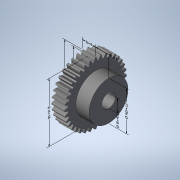
# Autodesk Inventor part: 29103600
Saved by Autodesk Inventor 2021 (Build 250183000, 183)
## iProperties
Created: 2026-04-15
Part Number: 29103600
Material: Generic
Catalog Web Link: www.3dfindit.com
Description: MAE-STZR-M0.5-POM-WS-Spur Gears Made from POM white, with One-Sided Hub, Module 0.5, Tooth Width 4 mm
Vendor: MAEDLER
Document SubType Name: Modeling
Designer: psAdmin
Manufacturer: MAEDLER
Mass: 1.8 g
Surface Area: 11.736 cm^2
Volume: 1.36263 cm^3
Density: 1 g/cm^3
Appearance: PSOLRGB-255-255-255
Category: PARTsolutions
Company: MAEDLER
Title: 29103600
Author: Cadenas PARTsolutions
Comments: Spur Gears Made from POM white, with One-Sided Hub, Module 0.5, Tooth Width 4 mm
PSOL_IDENT_0: {$CADENAS_DATA/23d-libs/maedler/antriebselemente/stirnzahnraeder/stirnzahnraeder_pom/stzr_pom_m_0_5.
PSOL_IDENT_1: prj},171 {VTYP=3D},{NB=29103600},{LINA=29103600},{NN=MAE-STZR-M0.5-POM-WS},{DATE=15.03.2026 14:49:43
PSOL_IDENT_2: },{GEOMDATE=15.03.2026 14:49:00},{VERSION=},{LINEID=220},{WBVAR=},{WBNUMERIC=}  {NB=29103600},{LINA=
PSOL_IDENT_3: 29103600},{KT=DUMMY},{ARTNR=29103600},{WEBSHOP=Produktdetails / Katalogseite / Montageanleitung},{MA
PSOL_IDENT_4: TK=Kunststoff weiß},{MAT=POM weiß},{M=0.5},{Z=36},{B=4},{DA=19.0},{D=18.0},{NL=4},{ND=12.0},{BJS10=4
PSOL_IDENT_5: },{MD=10.0},{GEW=1.80},{CTN=84839089},{DIST=0.900},{GKD=16.91447},{FKD=16.83300},{T0=1.57080},{UF=56
PSOL_IDENT_6: .54867},{TLG=1.57080},{A=3.07818},{A3=1.02606},{PI=0.39270},{R2=0.04},{CNSDWTEMPLATE=_dw/ansicht_rig
PSOL_IDENT_7: ht_front.dw}
NB: 29103600
NN: MAE-STZR-M0.5-POM-WS
NT: Spur Gears Made from POM white, with One-Sided Hub, Module 0.5, Tooth Width 4 mm
NBSYN: $ARTNR.
LINA: 29103600
CATALOG: MÄDLER
ARTNR: 29103600
WEBSHOP: Product details / Catalogue page / Assembly instructions
MATK: Plastic white
MAT: POM white
M: 0.5
Z: 36
B: 4
DA: 19
D: 18
NL: 4
ND: 12
BJS10: 4
MD: 10
GEW: 1.8
CTN: 84839089
SUPPLIER: MAEDLER
ARTICLENO: 29103600
BOMINFO: 29103600
CREATOR: CADENAS GmbH
Autodesk Inventor part; units mm, degrees
ref_plane "YZ Plane" through (0, 0, 0) normal (1, 0, 0) x (0, 1, 0)
ref_plane "XZ Plane" through (0, 0, 0) normal (0, 1, 0) x (-1, 0, 0)
ref_plane "XY Plane" through (0, 0, 0) normal (0, 0, 1) x (1, 0, 0)
sketch "Sketch_2" plane through (0, 0, 0) normal (0, 0, 1) x (1, 0, 0)
  line L0 (6, 0) -> (-2, 0)
  line L1 (-2, 9.5) -> (-2, 2.0707)
  line L2 (-2, 2.0707) -> (-1.9293, 2)
  line L3 (-1.9293, 2) -> (5.9293, 2)
  line L4 (5.9293, 2) -> (6, 2.0707)
  line L5 (6, 2.0707) -> (6, 5.9293)
  line L6 (6, 5.9293) -> (5.9293, 6)
  line L7 (5.9293, 6) -> (2.1, 6)
  arc A0 (2, 6.1) -> (2.1, 6) centre (2.1, 6.1) ccw
  line L8 (2, 6.1) -> (2, 9.5)
  line L9 (2, 9.5) -> (-2, 9.5)
  constraints: 20 end point, 2 point on circle, 1 centre point
revolve "Revolution1" add sketch "Sketch_2" angle 360 about axis through (6, 0, 0) along (1, 0, 0)
sketch "Sketch_4" plane through (0, 0, 0) normal (1, 0, 0) x (0, 0, -1)
  circle A0 centre (0, 0) radius 19
  arc A1 (-9.4982, 0.186) -> (-9.4982, -0.186) centre (0, 0) ccw
  arc A2 (-9.4982, -0.186) -> (-9.1353, -0.3433) centre (-7.9391, 2.9148) ccw
  arc A3 (-9.1353, -0.3433) -> (-8.9914, -0.3926) centre (-8.0658, 2.5431) ccw
  arc A4 (-8.9914, -0.3926) -> (-8.4349, -0.507) centre (-8.1752, 2.166) ccw
  arc A5 (-8.3989, -0.5443) -> (-8.4349, -0.507) centre (-8.4388, -0.5468) ccw
  arc A6 (-8.3989, -0.5443) -> (-8.3658, -0.9225) centre (0, 0) ccw
  arc A7 (-8.3948, -0.9654) -> (-8.3658, -0.9225) centre (-8.4056, -0.9268) ccw
  arc A8 (-8.3948, -0.9654) -> (-8.923, -1.1747) centre (-7.6749, -3.5527) ccw
  arc A9 (-8.923, -1.1747) -> (-9.0561, -1.2483) centre (-7.5017, -3.9051) ccw
  arc A10 (-9.0561, -1.2483) -> (-9.3862, -1.4661) centre (-7.3123, -4.2491) ccw
  arc A11 (-9.3862, -1.4661) -> (-9.3216, -1.8326) centre (0, 0) ccw
  arc A12 (-9.3216, -1.8326) -> (-8.9369, -1.9244) centre (-8.3246, 1.4919) ccw
  arc A13 (-8.9369, -1.9244) -> (-8.7867, -1.948) centre (-8.3849, 1.1039) ccw
  arc A14 (-8.7867, -1.948) -> (-8.2187, -1.964) centre (-8.4271, 0.7135) ccw
  arc A15 (-8.1768, -1.9944) -> (-8.2187, -1.964) centre (-8.2156, -2.0039) ccw
  arc A16 (-8.1768, -1.9944) -> (-8.0785, -2.3611) centre (0, 0) ccw
  arc A17 (-8.0997, -2.4085) -> (-8.0785, -2.3611) centre (-8.1169, -2.3724) ccw
  arc A18 (-8.0997, -2.4085) -> (-8.5835, -2.7064) centre (-6.9413, -4.8314) ccw
  arc A19 (-8.5835, -2.7064) -> (-8.7018, -2.8019) centre (-6.7096, -5.1484) ccw
  arc A20 (-8.7018, -2.8019) -> (-8.989, -3.0737) centre (-6.4633, -5.4544) ccw
  arc A21 (-8.989, -3.0737) -> (-8.8617, -3.4234) centre (0, 0) ccw
  arc A22 (-8.8617, -3.4234) -> (-8.4669, -3.447) centre (-8.4572, 0.0237) ccw
  arc A23 (-8.4669, -3.447) -> (-8.3149, -3.4442) centre (-8.4492, -0.3689) ccw
  arc A24 (-8.3149, -3.4442) -> (-7.7528, -3.3614) centre (-8.423, -0.7607) ccw
  arc A25 (-7.7062, -3.384) -> (-7.7528, -3.3614) centre (-7.7428, -3.4001) ccw
  arc A26 (-7.7062, -3.384) -> (-7.5458, -3.7281) centre (0, 0) ccw
  arc A27 (-7.5584, -3.7784) -> (-7.5458, -3.7281) centre (-7.5816, -3.7458) ccw
  arc A28 (-7.5584, -3.7784) -> (-7.9831, -4.1557) centre (-5.9969, -5.9634) ccw
  arc A29 (-7.9831, -4.1557) -> (-8.083, -4.2703) centre (-5.7136, -6.2353) ccw
  arc A30 (-8.083, -4.2703) -> (-8.3187, -4.588) centre (-5.418, -6.4938) ccw
  arc A31 (-8.3187, -4.588) -> (-8.1326, -4.9102) centre (0, 0) ccw
  arc A32 (-8.1326, -4.9102) -> (-7.7397, -4.8649) centre (-8.3328, -1.4452) ccw
  arc A33 (-7.7397, -4.8649) -> (-7.5905, -4.8357) centre (-8.2568, -1.8305) ccw
  arc A34 (-7.5905, -4.8357) -> (-7.0513, -4.6566) centre (-8.1629, -2.2118) ccw
  arc A35 (-7.0015, -4.6708) -> (-7.0513, -4.6566) centre (-7.0348, -4.693) ccw
  arc A36 (-7.0015, -4.6708) -> (-6.7838, -4.9818) centre (0, 0) ccw
  arc A37 (-6.7874, -5.0335) -> (-6.7838, -4.9818) centre (-6.816, -5.0054) ccw
  arc A38 (-6.7874, -5.0335) -> (-7.1402, -5.4789) centre (-4.8703, -6.9141) ccw
  arc A39 (-7.1402, -5.4789) -> (-7.2187, -5.6091) centre (-4.5441, -7.1328) ccw
  arc A40 (-7.2187, -5.6091) -> (-7.3956, -5.9628) centre (-4.2081, -7.336) ccw
  arc A41 (-7.3956, -5.9628) -> (-7.1564, -6.2478) centre (0, 0) ccw
  arc A42 (-7.1564, -6.2478) -> (-6.7774, -6.135) centre (-7.9553, -2.8702) ccw
  arc A43 (-6.7774, -6.135) -> (-6.6355, -6.0803) centre (-7.8135, -3.2364) ccw
  arc A44 (-6.6355, -6.0803) -> (-6.1356, -5.8103) centre (-7.6548, -3.5957) ccw
  arc A45 (-6.0841, -5.8156) -> (-6.1356, -5.8103) centre (-6.113, -5.8433) ccw
  arc A46 (-6.0841, -5.8156) -> (-5.8156, -6.0841) centre (0, 0) ccw
  arc A47 (-5.8103, -6.1356) -> (-5.8156, -6.0841) centre (-5.8433, -6.113) ccw
  arc A48 (-5.8103, -6.1356) -> (-6.0803, -6.6355) centre (-3.5957, -7.6548) ccw
  arc A49 (-6.0803, -6.6355) -> (-6.135, -6.7774) centre (-3.2364, -7.8135) ccw
  arc A50 (-6.135, -6.7774) -> (-6.2478, -7.1564) centre (-2.8702, -7.9553) ccw
  arc A51 (-6.2478, -7.1564) -> (-5.9628, -7.3956) centre (0, 0) ccw
  arc A52 (-5.9628, -7.3956) -> (-5.6091, -7.2187) centre (-7.336, -4.2081) ccw
  arc A53 (-5.6091, -7.2187) -> (-5.4789, -7.1402) centre (-7.1328, -4.5441) ccw
  arc A54 (-5.4789, -7.1402) -> (-5.0335, -6.7874) centre (-6.9141, -4.8703) ccw
  arc A55 (-4.9818, -6.7838) -> (-5.0335, -6.7874) centre (-5.0054, -6.816) ccw
  arc A56 (-4.9818, -6.7838) -> (-4.6708, -7.0015) centre (0, 0) ccw
  arc A57 (-4.6566, -7.0513) -> (-4.6708, -7.0015) centre (-4.693, -7.0348) ccw
  arc A58 (-4.6566, -7.0513) -> (-4.8357, -7.5905) centre (-2.2118, -8.1629) ccw
  arc A59 (-4.8357, -7.5905) -> (-4.8649, -7.7397) centre (-1.8305, -8.2568) ccw
  arc A60 (-4.8649, -7.7397) -> (-4.9102, -8.1326) centre (-1.4452, -8.3328) ccw
  arc A61 (-4.9102, -8.1326) -> (-4.588, -8.3187) centre (0, 0) ccw
  arc A62 (-4.588, -8.3187) -> (-4.2703, -8.083) centre (-6.4938, -5.418) ccw
  arc A63 (-4.2703, -8.083) -> (-4.1557, -7.9831) centre (-6.2353, -5.7136) ccw
  arc A64 (-4.1557, -7.9831) -> (-3.7784, -7.5584) centre (-5.9634, -5.9969) ccw
  arc A65 (-3.7281, -7.5458) -> (-3.7784, -7.5584) centre (-3.7458, -7.5816) ccw
  arc A66 (-3.7281, -7.5458) -> (-3.384, -7.7062) centre (0, 0) ccw
  arc A67 (-3.3614, -7.7528) -> (-3.384, -7.7062) centre (-3.4001, -7.7428) ccw
  arc A68 (-3.3614, -7.7528) -> (-3.4442, -8.3149) centre (-0.7607, -8.423) ccw
  arc A69 (-3.4442, -8.3149) -> (-3.447, -8.4669) centre (-0.3689, -8.4492) ccw
  arc A70 (-3.447, -8.4669) -> (-3.4234, -8.8617) centre (0.0237, -8.4572) ccw
  arc A71 (-3.4234, -8.8617) -> (-3.0737, -8.989) centre (0, 0) ccw
  arc A72 (-3.0737, -8.989) -> (-2.8019, -8.7018) centre (-5.4544, -6.4633) ccw
  arc A73 (-2.8019, -8.7018) -> (-2.7064, -8.5835) centre (-5.1484, -6.7096) ccw
  arc A74 (-2.7064, -8.5835) -> (-2.4085, -8.0997) centre (-4.8314, -6.9413) ccw
  arc A75 (-2.3611, -8.0785) -> (-2.4085, -8.0997) centre (-2.3724, -8.1169) ccw
  arc A76 (-2.3611, -8.0785) -> (-1.9944, -8.1768) centre (0, 0) ccw
  arc A77 (-1.964, -8.2187) -> (-1.9944, -8.1768) centre (-2.0039, -8.2156) ccw
  arc A78 (-1.964, -8.2187) -> (-1.948, -8.7867) centre (0.7135, -8.4271) ccw
  arc A79 (-1.948, -8.7867) -> (-1.9244, -8.9369) centre (1.1039, -8.3849) ccw
  arc A80 (-1.9244, -8.9369) -> (-1.8326, -9.3216) centre (1.4919, -8.3246) ccw
  arc A81 (-1.8326, -9.3216) -> (-1.4661, -9.3862) centre (0, 0) ccw
  arc A82 (-1.4661, -9.3862) -> (-1.2483, -9.0561) centre (-4.2491, -7.3123) ccw
  arc A83 (-1.2483, -9.0561) -> (-1.1747, -8.923) centre (-3.9051, -7.5017) ccw
  arc A84 (-1.1747, -8.923) -> (-0.9654, -8.3948) centre (-3.5527, -7.6749) ccw
  arc A85 (-0.9225, -8.3658) -> (-0.9654, -8.3948) centre (-0.9268, -8.4056) ccw
  arc A86 (-0.9225, -8.3658) -> (-0.5443, -8.3989) centre (0, 0) ccw
  arc A87 (-0.507, -8.4349) -> (-0.5443, -8.3989) centre (-0.5468, -8.4388) ccw
  arc A88 (-0.507, -8.4349) -> (-0.3926, -8.9914) centre (2.166, -8.1752) ccw
  arc A89 (-0.3926, -8.9914) -> (-0.3433, -9.1353) centre (2.5431, -8.0658) ccw
  arc A90 (-0.3433, -9.1353) -> (-0.186, -9.4982) centre (2.9148, -7.9391) ccw
  arc A91 (-0.186, -9.4982) -> (0.186, -9.4982) centre (0, 0) ccw
  arc A92 (0.186, -9.4982) -> (0.3433, -9.1353) centre (-2.9148, -7.9391) ccw
  arc A93 (0.3433, -9.1353) -> (0.3926, -8.9914) centre (-2.5431, -8.0658) ccw
  arc A94 (0.3926, -8.9914) -> (0.507, -8.4349) centre (-2.166, -8.1752) ccw
  arc A95 (0.5443, -8.3989) -> (0.507, -8.4349) centre (0.5468, -8.4388) ccw
  arc A96 (0.5443, -8.3989) -> (0.9225, -8.3658) centre (0, 0) ccw
  arc A97 (0.9654, -8.3948) -> (0.9225, -8.3658) centre (0.9268, -8.4056) ccw
  arc A98 (0.9654, -8.3948) -> (1.1747, -8.923) centre (3.5527, -7.6749) ccw
  arc A99 (1.1747, -8.923) -> (1.2483, -9.0561) centre (3.9051, -7.5017) ccw
  arc A100 (1.2483, -9.0561) -> (1.4661, -9.3862) centre (4.2491, -7.3123) ccw
  arc A101 (1.4661, -9.3862) -> (1.8326, -9.3216) centre (0, 0) ccw
  arc A102 (1.8326, -9.3216) -> (1.9244, -8.9369) centre (-1.4919, -8.3246) ccw
  arc A103 (1.9244, -8.9369) -> (1.948, -8.7867) centre (-1.1039, -8.3849) ccw
  arc A104 (1.948, -8.7867) -> (1.964, -8.2187) centre (-0.7135, -8.4271) ccw
  arc A105 (1.9944, -8.1768) -> (1.964, -8.2187) centre (2.0039, -8.2156) ccw
  arc A106 (1.9944, -8.1768) -> (2.3611, -8.0785) centre (0, 0) ccw
  arc A107 (2.4085, -8.0997) -> (2.3611, -8.0785) centre (2.3724, -8.1169) ccw
  arc A108 (2.4085, -8.0997) -> (2.7064, -8.5835) centre (4.8314, -6.9413) ccw
  arc A109 (2.7064, -8.5835) -> (2.8019, -8.7018) centre (5.1484, -6.7096) ccw
  arc A110 (2.8019, -8.7018) -> (3.0737, -8.989) centre (5.4544, -6.4633) ccw
  arc A111 (3.0737, -8.989) -> (3.4234, -8.8617) centre (0, 0) ccw
  arc A112 (3.4234, -8.8617) -> (3.447, -8.4669) centre (-0.0237, -8.4572) ccw
  arc A113 (3.447, -8.4669) -> (3.4442, -8.3149) centre (0.3689, -8.4492) ccw
  arc A114 (3.4442, -8.3149) -> (3.3614, -7.7528) centre (0.7607, -8.423) ccw
  arc A115 (3.384, -7.7062) -> (3.3614, -7.7528) centre (3.4001, -7.7428) ccw
  arc A116 (3.384, -7.7062) -> (3.7281, -7.5458) centre (0, 0) ccw
  arc A117 (3.7784, -7.5584) -> (3.7281, -7.5458) centre (3.7458, -7.5816) ccw
  arc A118 (3.7784, -7.5584) -> (4.1557, -7.9831) centre (5.9634, -5.9969) ccw
  arc A119 (4.1557, -7.9831) -> (4.2703, -8.083) centre (6.2353, -5.7136) ccw
  arc A120 (4.2703, -8.083) -> (4.588, -8.3187) centre (6.4938, -5.418) ccw
  arc A121 (4.588, -8.3187) -> (4.9102, -8.1326) centre (0, 0) ccw
  arc A122 (4.9102, -8.1326) -> (4.8649, -7.7397) centre (1.4452, -8.3328) ccw
  arc A123 (4.8649, -7.7397) -> (4.8357, -7.5905) centre (1.8305, -8.2568) ccw
  arc A124 (4.8357, -7.5905) -> (4.6566, -7.0513) centre (2.2118, -8.1629) ccw
  arc A125 (4.6708, -7.0015) -> (4.6566, -7.0513) centre (4.693, -7.0348) ccw
  arc A126 (4.6708, -7.0015) -> (4.9818, -6.7838) centre (0, 0) ccw
  arc A127 (5.0335, -6.7874) -> (4.9818, -6.7838) centre (5.0054, -6.816) ccw
  arc A128 (5.0335, -6.7874) -> (5.4789, -7.1402) centre (6.9141, -4.8703) ccw
  arc A129 (5.4789, -7.1402) -> (5.6091, -7.2187) centre (7.1328, -4.5441) ccw
  arc A130 (5.6091, -7.2187) -> (5.9628, -7.3956) centre (7.336, -4.2081) ccw
  arc A131 (5.9628, -7.3956) -> (6.2478, -7.1564) centre (0, 0) ccw
  arc A132 (6.2478, -7.1564) -> (6.135, -6.7774) centre (2.8702, -7.9553) ccw
  arc A133 (6.135, -6.7774) -> (6.0803, -6.6355) centre (3.2364, -7.8135) ccw
  arc A134 (6.0803, -6.6355) -> (5.8103, -6.1356) centre (3.5957, -7.6548) ccw
  arc A135 (5.8156, -6.0841) -> (5.8103, -6.1356) centre (5.8433, -6.113) ccw
  arc A136 (5.8156, -6.0841) -> (6.0841, -5.8156) centre (0, 0) ccw
  arc A137 (6.1356, -5.8103) -> (6.0841, -5.8156) centre (6.113, -5.8433) ccw
  arc A138 (6.1356, -5.8103) -> (6.6355, -6.0803) centre (7.6548, -3.5957) ccw
  arc A139 (6.6355, -6.0803) -> (6.7774, -6.135) centre (7.8135, -3.2364) ccw
  arc A140 (6.7774, -6.135) -> (7.1564, -6.2478) centre (7.9553, -2.8702) ccw
  arc A141 (7.1564, -6.2478) -> (7.3956, -5.9628) centre (0, 0) ccw
  arc A142 (7.3956, -5.9628) -> (7.2187, -5.6091) centre (4.2081, -7.336) ccw
  arc A143 (7.2187, -5.6091) -> (7.1402, -5.4789) centre (4.5441, -7.1328) ccw
  arc A144 (7.1402, -5.4789) -> (6.7874, -5.0335) centre (4.8703, -6.9141) ccw
  arc A145 (6.7838, -4.9818) -> (6.7874, -5.0335) centre (6.816, -5.0054) ccw
  arc A146 (6.7838, -4.9818) -> (7.0015, -4.6708) centre (0, 0) ccw
  arc A147 (7.0513, -4.6566) -> (7.0015, -4.6708) centre (7.0348, -4.693) ccw
  arc A148 (7.0513, -4.6566) -> (7.5905, -4.8357) centre (8.1629, -2.2118) ccw
  arc A149 (7.5905, -4.8357) -> (7.7397, -4.8649) centre (8.2568, -1.8305) ccw
  arc A150 (7.7397, -4.8649) -> (8.1326, -4.9102) centre (8.3328, -1.4452) ccw
  arc A151 (8.1326, -4.9102) -> (8.3187, -4.588) centre (0, 0) ccw
  arc A152 (8.3187, -4.588) -> (8.083, -4.2703) centre (5.418, -6.4938) ccw
  arc A153 (8.083, -4.2703) -> (7.9831, -4.1557) centre (5.7136, -6.2353) ccw
  arc A154 (7.9831, -4.1557) -> (7.5584, -3.7784) centre (5.9969, -5.9634) ccw
  arc A155 (7.5458, -3.7281) -> (7.5584, -3.7784) centre (7.5816, -3.7458) ccw
  arc A156 (7.5458, -3.7281) -> (7.7062, -3.384) centre (0, 0) ccw
  arc A157 (7.7528, -3.3614) -> (7.7062, -3.384) centre (7.7428, -3.4001) ccw
  arc A158 (7.7528, -3.3614) -> (8.3149, -3.4442) centre (8.423, -0.7607) ccw
  arc A159 (8.3149, -3.4442) -> (8.4669, -3.447) centre (8.4492, -0.3689) ccw
  arc A160 (8.4669, -3.447) -> (8.8617, -3.4234) centre (8.4572, 0.0237) ccw
  arc A161 (8.8617, -3.4234) -> (8.989, -3.0737) centre (0, 0) ccw
  arc A162 (8.989, -3.0737) -> (8.7018, -2.8019) centre (6.4633, -5.4544) ccw
  arc A163 (8.7018, -2.8019) -> (8.5835, -2.7064) centre (6.7096, -5.1484) ccw
  arc A164 (8.5835, -2.7064) -> (8.0997, -2.4085) centre (6.9413, -4.8314) ccw
  arc A165 (8.0785, -2.3611) -> (8.0997, -2.4085) centre (8.1169, -2.3724) ccw
  arc A166 (8.0785, -2.3611) -> (8.1768, -1.9944) centre (0, 0) ccw
  arc A167 (8.2187, -1.964) -> (8.1768, -1.9944) centre (8.2156, -2.0039) ccw
  arc A168 (8.2187, -1.964) -> (8.7867, -1.948) centre (8.4271, 0.7135) ccw
  arc A169 (8.7867, -1.948) -> (8.9369, -1.9244) centre (8.3849, 1.1039) ccw
  arc A170 (8.9369, -1.9244) -> (9.3216, -1.8326) centre (8.3246, 1.4919) ccw
  arc A171 (9.3216, -1.8326) -> (9.3862, -1.4661) centre (0, 0) ccw
  arc A172 (9.3862, -1.4661) -> (9.0561, -1.2483) centre (7.3123, -4.2491) ccw
  arc A173 (9.0561, -1.2483) -> (8.923, -1.1747) centre (7.5017, -3.9051) ccw
  arc A174 (8.923, -1.1747) -> (8.3948, -0.9654) centre (7.6749, -3.5527) ccw
  arc A175 (8.3658, -0.9225) -> (8.3948, -0.9654) centre (8.4056, -0.9268) ccw
  arc A176 (8.3658, -0.9225) -> (8.3989, -0.5443) centre (0, 0) ccw
  arc A177 (8.4349, -0.507) -> (8.3989, -0.5443) centre (8.4388, -0.5468) ccw
  arc A178 (8.4349, -0.507) -> (8.9914, -0.3926) centre (8.1752, 2.166) ccw
  arc A179 (8.9914, -0.3926) -> (9.1353, -0.3433) centre (8.0658, 2.5431) ccw
  arc A180 (9.1353, -0.3433) -> (9.4982, -0.186) centre (7.9391, 2.9148) ccw
  arc A181 (9.4982, -0.186) -> (9.4982, 0.186) centre (0, 0) ccw
  arc A182 (9.4982, 0.186) -> (9.1353, 0.3433) centre (7.9391, -2.9148) ccw
  arc A183 (9.1353, 0.3433) -> (8.9914, 0.3926) centre (8.0658, -2.5431) ccw
  arc A184 (8.9914, 0.3926) -> (8.4349, 0.507) centre (8.1752, -2.166) ccw
  arc A185 (8.3989, 0.5443) -> (8.4349, 0.507) centre (8.4388, 0.5468) ccw
  arc A186 (8.3989, 0.5443) -> (8.3658, 0.9225) centre (0, 0) ccw
  arc A187 (8.3948, 0.9654) -> (8.3658, 0.9225) centre (8.4056, 0.9268) ccw
  arc A188 (8.3948, 0.9654) -> (8.923, 1.1747) centre (7.6749, 3.5527) ccw
  arc A189 (8.923, 1.1747) -> (9.0561, 1.2483) centre (7.5017, 3.9051) ccw
  arc A190 (9.0561, 1.2483) -> (9.3862, 1.4661) centre (7.3123, 4.2491) ccw
  arc A191 (9.3862, 1.4661) -> (9.3216, 1.8326) centre (0, 0) ccw
  arc A192 (9.3216, 1.8326) -> (8.9369, 1.9244) centre (8.3246, -1.4919) ccw
  arc A193 (8.9369, 1.9244) -> (8.7867, 1.948) centre (8.3849, -1.1039) ccw
  arc A194 (8.7867, 1.948) -> (8.2187, 1.964) centre (8.4271, -0.7135) ccw
  arc A195 (8.1768, 1.9944) -> (8.2187, 1.964) centre (8.2156, 2.0039) ccw
  arc A196 (8.1768, 1.9944) -> (8.0785, 2.3611) centre (0, 0) ccw
  arc A197 (8.0997, 2.4085) -> (8.0785, 2.3611) centre (8.1169, 2.3724) ccw
  arc A198 (8.0997, 2.4085) -> (8.5835, 2.7064) centre (6.9413, 4.8314) ccw
  arc A199 (8.5835, 2.7064) -> (8.7018, 2.8019) centre (6.7096, 5.1484) ccw
  arc A200 (8.7018, 2.8019) -> (8.989, 3.0737) centre (6.4633, 5.4544) ccw
  arc A201 (8.989, 3.0737) -> (8.8617, 3.4234) centre (0, 0) ccw
  arc A202 (8.8617, 3.4234) -> (8.4669, 3.447) centre (8.4572, -0.0237) ccw
  arc A203 (8.4669, 3.447) -> (8.3149, 3.4442) centre (8.4492, 0.3689) ccw
  arc A204 (8.3149, 3.4442) -> (7.7528, 3.3614) centre (8.423, 0.7607) ccw
  arc A205 (7.7062, 3.384) -> (7.7528, 3.3614) centre (7.7428, 3.4001) ccw
  arc A206 (7.7062, 3.384) -> (7.5458, 3.7281) centre (0, 0) ccw
  arc A207 (7.5584, 3.7784) -> (7.5458, 3.7281) centre (7.5816, 3.7458) ccw
  arc A208 (7.5584, 3.7784) -> (7.9831, 4.1557) centre (5.9969, 5.9634) ccw
  arc A209 (7.9831, 4.1557) -> (8.083, 4.2703) centre (5.7136, 6.2353) ccw
  arc A210 (8.083, 4.2703) -> (8.3187, 4.588) centre (5.418, 6.4938) ccw
  arc A211 (8.3187, 4.588) -> (8.1326, 4.9102) centre (0, 0) ccw
  arc A212 (8.1326, 4.9102) -> (7.7397, 4.8649) centre (8.3328, 1.4452) ccw
  arc A213 (7.7397, 4.8649) -> (7.5905, 4.8357) centre (8.2568, 1.8305) ccw
  arc A214 (7.5905, 4.8357) -> (7.0513, 4.6566) centre (8.1629, 2.2118) ccw
  arc A215 (7.0015, 4.6708) -> (7.0513, 4.6566) centre (7.0348, 4.693) ccw
  arc A216 (7.0015, 4.6708) -> (6.7838, 4.9818) centre (0, 0) ccw
  arc A217 (6.7874, 5.0335) -> (6.7838, 4.9818) centre (6.816, 5.0054) ccw
  arc A218 (6.7874, 5.0335) -> (7.1402, 5.4789) centre (4.8703, 6.9141) ccw
  arc A219 (7.1402, 5.4789) -> (7.2187, 5.6091) centre (4.5441, 7.1328) ccw
  arc A220 (7.2187, 5.6091) -> (7.3956, 5.9628) centre (4.2081, 7.336) ccw
  arc A221 (7.3956, 5.9628) -> (7.1564, 6.2478) centre (0, 0) ccw
  arc A222 (7.1564, 6.2478) -> (6.7774, 6.135) centre (7.9553, 2.8702) ccw
  arc A223 (6.7774, 6.135) -> (6.6355, 6.0803) centre (7.8135, 3.2364) ccw
  arc A224 (6.6355, 6.0803) -> (6.1356, 5.8103) centre (7.6548, 3.5957) ccw
  arc A225 (6.0841, 5.8156) -> (6.1356, 5.8103) centre (6.113, 5.8433) ccw
  arc A226 (6.0841, 5.8156) -> (5.8156, 6.0841) centre (0, 0) ccw
  arc A227 (5.8103, 6.1356) -> (5.8156, 6.0841) centre (5.8433, 6.113) ccw
  arc A228 (5.8103, 6.1356) -> (6.0803, 6.6355) centre (3.5957, 7.6548) ccw
  arc A229 (6.0803, 6.6355) -> (6.135, 6.7774) centre (3.2364, 7.8135) ccw
  arc A230 (6.135, 6.7774) -> (6.2478, 7.1564) centre (2.8702, 7.9553) ccw
  arc A231 (6.2478, 7.1564) -> (5.9628, 7.3956) centre (0, 0) ccw
  arc A232 (5.9628, 7.3956) -> (5.6091, 7.2187) centre (7.336, 4.2081) ccw
  arc A233 (5.6091, 7.2187) -> (5.4789, 7.1402) centre (7.1328, 4.5441) ccw
  arc A234 (5.4789, 7.1402) -> (5.0335, 6.7874) centre (6.9141, 4.8703) ccw
  arc A235 (4.9818, 6.7838) -> (5.0335, 6.7874) centre (5.0054, 6.816) ccw
  arc A236 (4.9818, 6.7838) -> (4.6708, 7.0015) centre (0, 0) ccw
  arc A237 (4.6566, 7.0513) -> (4.6708, 7.0015) centre (4.693, 7.0348) ccw
  arc A238 (4.6566, 7.0513) -> (4.8357, 7.5905) centre (2.2118, 8.1629) ccw
  arc A239 (4.8357, 7.5905) -> (4.8649, 7.7397) centre (1.8305, 8.2568) ccw
  arc A240 (4.8649, 7.7397) -> (4.9102, 8.1326) centre (1.4452, 8.3328) ccw
  arc A241 (4.9102, 8.1326) -> (4.588, 8.3187) centre (0, 0) ccw
  arc A242 (4.588, 8.3187) -> (4.2703, 8.083) centre (6.4938, 5.418) ccw
  arc A243 (4.2703, 8.083) -> (4.1557, 7.9831) centre (6.2353, 5.7136) ccw
  arc A244 (4.1557, 7.9831) -> (3.7784, 7.5584) centre (5.9634, 5.9969) ccw
  arc A245 (3.7281, 7.5458) -> (3.7784, 7.5584) centre (3.7458, 7.5816) ccw
  arc A246 (3.7281, 7.5458) -> (3.384, 7.7062) centre (0, 0) ccw
  arc A247 (3.3614, 7.7528) -> (3.384, 7.7062) centre (3.4001, 7.7428) ccw
  arc A248 (3.3614, 7.7528) -> (3.4442, 8.3149) centre (0.7607, 8.423) ccw
  arc A249 (3.4442, 8.3149) -> (3.447, 8.4669) centre (0.3689, 8.4492) ccw
  arc A250 (3.447, 8.4669) -> (3.4234, 8.8617) centre (-0.0237, 8.4572) ccw
  arc A251 (3.4234, 8.8617) -> (3.0737, 8.989) centre (0, 0) ccw
  arc A252 (3.0737, 8.989) -> (2.8019, 8.7018) centre (5.4544, 6.4633) ccw
  arc A253 (2.8019, 8.7018) -> (2.7064, 8.5835) centre (5.1484, 6.7096) ccw
  arc A254 (2.7064, 8.5835) -> (2.4085, 8.0997) centre (4.8314, 6.9413) ccw
  arc A255 (2.3611, 8.0785) -> (2.4085, 8.0997) centre (2.3724, 8.1169) ccw
  arc A256 (2.3611, 8.0785) -> (1.9944, 8.1768) centre (0, 0) ccw
  arc A257 (1.964, 8.2187) -> (1.9944, 8.1768) centre (2.0039, 8.2156) ccw
  arc A258 (1.964, 8.2187) -> (1.948, 8.7867) centre (-0.7135, 8.4271) ccw
  arc A259 (1.948, 8.7867) -> (1.9244, 8.9369) centre (-1.1039, 8.3849) ccw
  arc A260 (1.9244, 8.9369) -> (1.8326, 9.3216) centre (-1.4919, 8.3246) ccw
  arc A261 (1.8326, 9.3216) -> (1.4661, 9.3862) centre (0, 0) ccw
  arc A262 (1.4661, 9.3862) -> (1.2483, 9.0561) centre (4.2491, 7.3123) ccw
  arc A263 (1.2483, 9.0561) -> (1.1747, 8.923) centre (3.9051, 7.5017) ccw
  arc A264 (1.1747, 8.923) -> (0.9654, 8.3948) centre (3.5527, 7.6749) ccw
  arc A265 (0.9225, 8.3658) -> (0.9654, 8.3948) centre (0.9268, 8.4056) ccw
  arc A266 (0.9225, 8.3658) -> (0.5443, 8.3989) centre (0, 0) ccw
  arc A267 (0.507, 8.4349) -> (0.5443, 8.3989) centre (0.5468, 8.4388) ccw
  arc A268 (0.507, 8.4349) -> (0.3926, 8.9914) centre (-2.166, 8.1752) ccw
  arc A269 (0.3926, 8.9914) -> (0.3433, 9.1353) centre (-2.5431, 8.0658) ccw
  arc A270 (0.3433, 9.1353) -> (0.186, 9.4982) centre (-2.9148, 7.9391) ccw
  arc A271 (0.186, 9.4982) -> (-0.186, 9.4982) centre (0, 0) ccw
  arc A272 (-0.186, 9.4982) -> (-0.3433, 9.1353) centre (2.9148, 7.9391) ccw
  arc A273 (-0.3433, 9.1353) -> (-0.3926, 8.9914) centre (2.5431, 8.0658) ccw
  arc A274 (-0.3926, 8.9914) -> (-0.507, 8.4349) centre (2.166, 8.1752) ccw
  arc A275 (-0.5443, 8.3989) -> (-0.507, 8.4349) centre (-0.5468, 8.4388) ccw
  arc A276 (-0.5443, 8.3989) -> (-0.9225, 8.3658) centre (0, 0) ccw
  arc A277 (-0.9654, 8.3948) -> (-0.9225, 8.3658) centre (-0.9268, 8.4056) ccw
  arc A278 (-0.9654, 8.3948) -> (-1.1747, 8.923) centre (-3.5527, 7.6749) ccw
  arc A279 (-1.1747, 8.923) -> (-1.2483, 9.0561) centre (-3.9051, 7.5017) ccw
  arc A280 (-1.2483, 9.0561) -> (-1.4661, 9.3862) centre (-4.2491, 7.3123) ccw
  arc A281 (-1.4661, 9.3862) -> (-1.8326, 9.3216) centre (0, 0) ccw
  arc A282 (-1.8326, 9.3216) -> (-1.9244, 8.9369) centre (1.4919, 8.3246) ccw
  arc A283 (-1.9244, 8.9369) -> (-1.948, 8.7867) centre (1.1039, 8.3849) ccw
  arc A284 (-1.948, 8.7867) -> (-1.964, 8.2187) centre (0.7135, 8.4271) ccw
  arc A285 (-1.9944, 8.1768) -> (-1.964, 8.2187) centre (-2.0039, 8.2156) ccw
  arc A286 (-1.9944, 8.1768) -> (-2.3611, 8.0785) centre (0, 0) ccw
  arc A287 (-2.4085, 8.0997) -> (-2.3611, 8.0785) centre (-2.3724, 8.1169) ccw
  arc A288 (-2.4085, 8.0997) -> (-2.7064, 8.5835) centre (-4.8314, 6.9413) ccw
  arc A289 (-2.7064, 8.5835) -> (-2.8019, 8.7018) centre (-5.1484, 6.7096) ccw
  arc A290 (-2.8019, 8.7018) -> (-3.0737, 8.989) centre (-5.4544, 6.4633) ccw
  arc A291 (-3.0737, 8.989) -> (-3.4234, 8.8617) centre (0, 0) ccw
  arc A292 (-3.4234, 8.8617) -> (-3.447, 8.4669) centre (0.0237, 8.4572) ccw
  arc A293 (-3.447, 8.4669) -> (-3.4442, 8.3149) centre (-0.3689, 8.4492) ccw
  arc A294 (-3.4442, 8.3149) -> (-3.3614, 7.7528) centre (-0.7607, 8.423) ccw
  arc A295 (-3.384, 7.7062) -> (-3.3614, 7.7528) centre (-3.4001, 7.7428) ccw
  arc A296 (-3.384, 7.7062) -> (-3.7281, 7.5458) centre (0, 0) ccw
  arc A297 (-3.7784, 7.5584) -> (-3.7281, 7.5458) centre (-3.7458, 7.5816) ccw
  arc A298 (-3.7784, 7.5584) -> (-4.1557, 7.9831) centre (-5.9634, 5.9969) ccw
  arc A299 (-4.1557, 7.9831) -> (-4.2703, 8.083) centre (-6.2353, 5.7136) ccw
  arc A300 (-4.2703, 8.083) -> (-4.588, 8.3187) centre (-6.4938, 5.418) ccw
  arc A301 (-4.588, 8.3187) -> (-4.9102, 8.1326) centre (0, 0) ccw
  arc A302 (-4.9102, 8.1326) -> (-4.8649, 7.7397) centre (-1.4452, 8.3328) ccw
  arc A303 (-4.8649, 7.7397) -> (-4.8357, 7.5905) centre (-1.8305, 8.2568) ccw
  arc A304 (-4.8357, 7.5905) -> (-4.6566, 7.0513) centre (-2.2118, 8.1629) ccw
  arc A305 (-4.6708, 7.0015) -> (-4.6566, 7.0513) centre (-4.693, 7.0348) ccw
  arc A306 (-4.6708, 7.0015) -> (-4.9818, 6.7838) centre (0, 0) ccw
  arc A307 (-5.0335, 6.7874) -> (-4.9818, 6.7838) centre (-5.0054, 6.816) ccw
  arc A308 (-5.0335, 6.7874) -> (-5.4789, 7.1402) centre (-6.9141, 4.8703) ccw
  arc A309 (-5.4789, 7.1402) -> (-5.6091, 7.2187) centre (-7.1328, 4.5441) ccw
  arc A310 (-5.6091, 7.2187) -> (-5.9628, 7.3956) centre (-7.336, 4.2081) ccw
  arc A311 (-5.9628, 7.3956) -> (-6.2478, 7.1564) centre (0, 0) ccw
  arc A312 (-6.2478, 7.1564) -> (-6.135, 6.7774) centre (-2.8702, 7.9553) ccw
  arc A313 (-6.135, 6.7774) -> (-6.0803, 6.6355) centre (-3.2364, 7.8135) ccw
  arc A314 (-6.0803, 6.6355) -> (-5.8103, 6.1356) centre (-3.5957, 7.6548) ccw
  arc A315 (-5.8156, 6.0841) -> (-5.8103, 6.1356) centre (-5.8433, 6.113) ccw
  arc A316 (-5.8156, 6.0841) -> (-6.0841, 5.8156) centre (0, 0) ccw
  arc A317 (-6.1356, 5.8103) -> (-6.0841, 5.8156) centre (-6.113, 5.8433) ccw
  arc A318 (-6.1356, 5.8103) -> (-6.6355, 6.0803) centre (-7.6548, 3.5957) ccw
  arc A319 (-6.6355, 6.0803) -> (-6.7774, 6.135) centre (-7.8135, 3.2364) ccw
  arc A320 (-6.7774, 6.135) -> (-7.1564, 6.2478) centre (-7.9553, 2.8702) ccw
  arc A321 (-7.1564, 6.2478) -> (-7.3956, 5.9628) centre (0, 0) ccw
  arc A322 (-7.3956, 5.9628) -> (-7.2187, 5.6091) centre (-4.2081, 7.336) ccw
  arc A323 (-7.2187, 5.6091) -> (-7.1402, 5.4789) centre (-4.5441, 7.1328) ccw
  arc A324 (-7.1402, 5.4789) -> (-6.7874, 5.0335) centre (-4.8703, 6.9141) ccw
  arc A325 (-6.7838, 4.9818) -> (-6.7874, 5.0335) centre (-6.816, 5.0054) ccw
  arc A326 (-6.7838, 4.9818) -> (-7.0015, 4.6708) centre (0, 0) ccw
  arc A327 (-7.0513, 4.6566) -> (-7.0015, 4.6708) centre (-7.0348, 4.693) ccw
  arc A328 (-7.0513, 4.6566) -> (-7.5905, 4.8357) centre (-8.1629, 2.2118) ccw
  arc A329 (-7.5905, 4.8357) -> (-7.7397, 4.8649) centre (-8.2568, 1.8305) ccw
  arc A330 (-7.7397, 4.8649) -> (-8.1326, 4.9102) centre (-8.3328, 1.4452) ccw
  arc A331 (-8.1326, 4.9102) -> (-8.3187, 4.588) centre (0, 0) ccw
  arc A332 (-8.3187, 4.588) -> (-8.083, 4.2703) centre (-5.418, 6.4938) ccw
  arc A333 (-8.083, 4.2703) -> (-7.9831, 4.1557) centre (-5.7136, 6.2353) ccw
  arc A334 (-7.9831, 4.1557) -> (-7.5584, 3.7784) centre (-5.9969, 5.9634) ccw
  arc A335 (-7.5458, 3.7281) -> (-7.5584, 3.7784) centre (-7.5816, 3.7458) ccw
  arc A336 (-7.5458, 3.7281) -> (-7.7062, 3.384) centre (0, 0) ccw
  arc A337 (-7.7528, 3.3614) -> (-7.7062, 3.384) centre (-7.7428, 3.4001) ccw
  arc A338 (-7.7528, 3.3614) -> (-8.3149, 3.4442) centre (-8.423, 0.7607) ccw
  arc A339 (-8.3149, 3.4442) -> (-8.4669, 3.447) centre (-8.4492, 0.3689) ccw
  arc A340 (-8.4669, 3.447) -> (-8.8617, 3.4234) centre (-8.4572, -0.0237) ccw
  arc A341 (-8.8617, 3.4234) -> (-8.989, 3.0737) centre (0, 0) ccw
  arc A342 (-8.989, 3.0737) -> (-8.7018, 2.8019) centre (-6.4633, 5.4544) ccw
  arc A343 (-8.7018, 2.8019) -> (-8.5835, 2.7064) centre (-6.7096, 5.1484) ccw
  arc A344 (-8.5835, 2.7064) -> (-8.0997, 2.4085) centre (-6.9413, 4.8314) ccw
  arc A345 (-8.0785, 2.3611) -> (-8.0997, 2.4085) centre (-8.1169, 2.3724) ccw
  arc A346 (-8.0785, 2.3611) -> (-8.1768, 1.9944) centre (0, 0) ccw
  arc A347 (-8.2187, 1.964) -> (-8.1768, 1.9944) centre (-8.2156, 2.0039) ccw
  arc A348 (-8.2187, 1.964) -> (-8.7867, 1.948) centre (-8.4271, -0.7135) ccw
  arc A349 (-8.7867, 1.948) -> (-8.9369, 1.9244) centre (-8.3849, -1.1039) ccw
  arc A350 (-8.9369, 1.9244) -> (-9.3216, 1.8326) centre (-8.3246, -1.4919) ccw
  arc A351 (-9.3216, 1.8326) -> (-9.3862, 1.4661) centre (0, 0) ccw
  arc A352 (-9.3862, 1.4661) -> (-9.0561, 1.2483) centre (-7.3123, 4.2491) ccw
  arc A353 (-9.0561, 1.2483) -> (-8.923, 1.1747) centre (-7.5017, 3.9051) ccw
  arc A354 (-8.923, 1.1747) -> (-8.3948, 0.9654) centre (-7.6749, 3.5527) ccw
  arc A355 (-8.3658, 0.9225) -> (-8.3948, 0.9654) centre (-8.4056, 0.9268) ccw
  arc A356 (-8.3658, 0.9225) -> (-8.3989, 0.5443) centre (0, 0) ccw
  arc A357 (-8.4349, 0.507) -> (-8.3989, 0.5443) centre (-8.4388, 0.5468) ccw
  arc A358 (-8.4349, 0.507) -> (-8.9914, 0.3926) centre (-8.1752, -2.166) ccw
  arc A359 (-8.9914, 0.3926) -> (-9.1353, 0.3433) centre (-8.0658, -2.5431) ccw
  arc A360 (-9.1353, 0.3433) -> (-9.4982, 0.186) centre (-7.9391, -2.9148) ccw
  constraints: 720 point on circle, 361 centre point
extrude "Extrusion1" cut sketch "Sketch_4" along normal mid plane 4
body "Solid1"
